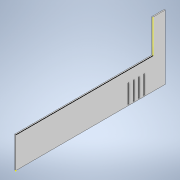
# Autodesk Inventor part: 220207 Right Side
Saved by Autodesk Inventor 2022 (Build 260153000, 153)
## iProperties
Created: 2022-02-07
Part Number: 220207 Right Side
Material: Generic
Document SubType Name: Modeling
Designer: josephinew
Density: 1 g/cm^3
Appearance: Default
Author: josephinew
Autodesk Inventor part; units mm, degrees
ref_plane "YZ Plane" through (0, 0, 0) normal (1, 0, 0) x (0, 1, 0)
ref_plane "XZ Plane" through (0, 0, 0) normal (0, 1, 0) x (-1, 0, 0)
ref_plane "XY Plane" through (0, 0, 0) normal (0, 0, 1) x (1, 0, 0)
sketch "Sketch1" plane through (0, 0, 0) normal (1, 0, 0) x (0, 1, 0)
  line L0 (0, 0) -> (95.25, 0)
  line L1 (95.25, 0) -> (95.25, -419.1)
  line L2 (95.25, -457.2) -> (0, -457.2)
  line L3 (0, -457.2) -> (0, 0)
  line L4 (0, -457.2) -> (196.85, -457.2)
  line L5 (196.85, -457.2) -> (196.85, -419.1)
  line L6 (196.85, -419.1) -> (95.25, -419.1)
  line L7 (0, -419.1) -> (0, -457.2)
  constraints: 16 end point, 4 parallel, 2 horizontal, 2 perpendicular
extrude "Extrusion1" add sketch "Sketch1" along normal blind 3.175
sketch "Sketch2" plane through (3.175, 0, 0) normal (1, 0, 0) x (0, 0, -1)
  line L0 (393.7, 60.325) -> (390.525, 60.325)
  line L1 (377.825, 60.325) -> (374.65, 60.325)
  line L2 (361.95, 60.325) -> (358.775, 60.325)
  line L3 (346.075, 60.325) -> (342.9, 60.325)
  line L4 (342.9, 60.325) -> (342.9, 3.175)
  line L5 (358.775, 60.325) -> (358.775, 3.175)
  line L6 (346.075, 3.175) -> (346.075, 60.325)
  line L7 (361.95, 3.175) -> (361.95, 60.325)
  line L8 (361.95, 60.325) -> (358.775, 60.325)
  line L9 (358.775, 60.325) -> (358.775, 3.175)
  line L10 (361.95, 60.325) -> (361.95, 3.175)
  line L11 (374.65, 3.175) -> (374.65, 60.325)
  line L12 (377.825, 3.175) -> (377.825, 60.325)
  line L13 (377.825, 60.325) -> (374.65, 60.325)
  line L14 (374.65, 60.325) -> (374.65, 3.175)
  line L15 (377.825, 60.325) -> (377.825, 3.175)
  line L16 (390.525, 3.175) -> (390.525, 60.325)
  line L17 (393.7, 3.175) -> (393.7, 60.325)
  line L18 (393.7, 60.325) -> (390.525, 60.325)
  line L19 (390.525, 60.325) -> (390.525, 3.175)
  line L20 (346.075, 3.175) -> (342.9, 3.175)
  line L21 (342.9, 3.175) -> (346.075, 3.175)
  line L22 (358.775, 3.175) -> (361.95, 3.175)
  line L23 (374.65, 3.175) -> (377.825, 3.175)
  line L24 (390.525, 3.175) -> (393.7, 3.175)
  line L25 (419.1, 95.25) -> (0, 95.25) projected
  line L26 (0, 95.25) -> (457.2, 95.25)
  line L27 (457.2, 95.25) -> (457.2, 0)
  line L28 (457.2, 0) -> (0, 0)
  line L29 (0, 0) -> (0, 95.25)
  constraints: 58 end point, 2 parallel, 1 horizontal, 1 perpendicular
extrude "Extrusion2" cut sketch "Sketch2" against normal blind 25.4 contours L17 L24 L16 L0 | L12 L23 L11 L1 | L7 L22 L5 L2 | L6 L20 L4 L3
sketch "Sketch3" plane through (3.175, 0, 0) normal (1, 0, 0) x (0, 0, -1)
  point P0 (0, 0)
sketch "Sketch4" plane through (3.175, 0, 0) normal (1, 0, 0) x (0, 0, -1)
  point P0 (0, 0)
sketch "Sketch5" plane through (3.175, 0, 0) normal (1, 0, 0) x (0, 0, -1)
  line L0 (419.1, 196.85) -> (419.1, 95.25) projected
  line L1 (419.1, 95.25) -> (0, 95.25) projected
  line L2 (419.1, 95.25) -> (0, 95.25)
  point P0 (0, 0)
  constraints: 2 end point, 1 collinear
body "Solid1"
